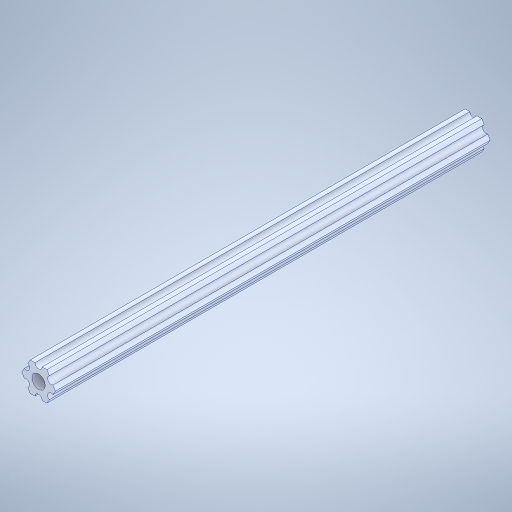
# Autodesk Inventor part: Main_churro
Saved by Autodesk Inventor 2023 (Build 270158000, 158)
## iProperties
Created: 2016-04-18
Part Number: Main_churro
Material: Generic
Description: STEP AP214
Document SubType Name: Modeling
Designer: jackc
Density: 1 g/cm^3
Appearance: Default
Sending System: SolidWorks 2014
Preprocessor: SwSTEP 2.0
Title: am-churro 500 churro tube.STEP
Revision Number: ANY
Autodesk Inventor part; units mm, degrees
ref_plane "YZ Plane" through (0, 0, 0) normal (1, 0, 0) x (0, 1, 0)
ref_plane "XZ Plane" through (0, 0, 0) normal (0, 1, 0) x (-1, 0, 0)
ref_plane "XY Plane" through (0, 0, 0) normal (0, 0, 1) x (1, 0, 0)
ref_plane "Work Plane1" through (0, 6.35, 304.8) normal (0, 0, 1) x (1, 0.0000001, 0)
sketch "Sketch1" plane through (0, 6.35, 304.8) normal (0, 0, 1) x (1, 0.0000001, 0)
  line L0 (6.293, -8.1502) -> (7.3323, -6.35) projected
  line L1 (7.3323, -6.35) -> (6.293, -4.5498) projected
  arc A0 (4.7055, -1.8002) -> (6.293, -4.5498) centre (5.4993, -3.175) ccw projected
  line L2 (4.7055, -1.8002) -> (3.6662, 0) projected
  line L3 (3.6662, 0) -> (1.5875, 0) projected
  arc A1 (-1.5875, 0) -> (1.5875, 0) centre (0, 0) ccw projected
  line L4 (-1.5875, 0) -> (-3.6662, 0) projected
  line L5 (-3.6662, 0) -> (-4.7055, -1.8002) projected
  arc A2 (-6.293, -4.5498) -> (-4.7055, -1.8002) centre (-5.4993, -3.175) ccw projected
  line L6 (-6.293, -4.5498) -> (-7.3323, -6.35) projected
  line L7 (-7.3323, -6.35) -> (-6.293, -8.1502) projected
  arc A3 (-4.7055, -10.8998) -> (-6.293, -8.1502) centre (-5.4993, -9.525) ccw projected
  line L8 (-4.7055, -10.8998) -> (-3.6662, -12.7) projected
  line L9 (-3.6662, -12.7) -> (-1.5875, -12.7) projected
  arc A4 (1.5875, -12.7) -> (-1.5875, -12.7) centre (0, -12.7) ccw projected
  line L10 (1.5875, -12.7) -> (3.6662, -12.7) projected
  line L11 (3.6662, -12.7) -> (4.7055, -10.8998) projected
  arc A5 (6.293, -8.1502) -> (4.7055, -10.8998) centre (5.4993, -9.525) ccw projected
  circle A6 centre (0, -6.35) radius 2.9337 projected
extrude "Extrusion1" add sketch "Sketch1" along normal blind 190.5
body "Solid2"
